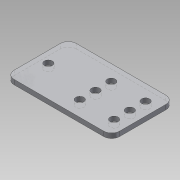
# Autodesk Inventor part: VSlot Idler Pulley Plate
Saved by Autodesk Inventor 2016 (Build 200138000, 138)
## iProperties
Created: 2013-06-20
Part Number: VSlot Idler Pulley Plate
Material: Aluminum 6061
Document SubType Name: Modeling
Designer: Jon Hollander
Density: 2.71 g/cm^3
Mass: 20.179 g
Surface Area: 59.138 cm^2
Volume: 7.44613 cm^3
Appearance: Aluminum - Flat
Author: Jon Hollander
Autodesk Inventor part; units mm, degrees
ref_plane "YZ Plane" through (0, 0, 0) normal (1, 0, 0) x (0, 1, 0)
ref_plane "XZ Plane" through (0, 0, 0) normal (0, 1, 0) x (-1, 0, 0)
ref_plane "XY Plane" through (0, 0, 0) normal (0, 0, 1) x (1, 0, 0)
sketch "Sketch2" plane through (0, 0, 0) normal (0, 0, 1) x (1, 0, 0)
  line L0 (-33.5, 19.75) -> (33.5, 19.75)
  line L1 (33.5, 19.75) -> (33.5, -19.75)
  line L2 (33.5, -19.75) -> (-33.5, -19.75)
  line L3 (-33.5, -19.75) -> (-33.5, 19.75)
  line L4 (-33.5, 19.75) -> (33.5, -19.75) construction
  line L5 (33.5, 19.75) -> (-33.5, -19.75) construction
  point P0 (0, 0)
  dimension "d0" = 67
  dimension "d1" = 39.5
  constraints: 12 end point, 2 midpoint, 2 parallel, 1 horizontal, 1 perpendicular
  measures "d0" distance of L1.end L2.end
  measures "d1" distance of L0.end L1.end
extrude "Extrusion1" add sketch "Sketch2" along normal blind 3
sketch "Sketch3" plane through (0, 0, 3) normal (0, 0, 1) x (1, 0, 0)
  line L0 (33.5, 19.75) -> (-33.5, 19.75) projected
  line L1 (-33.5, 19.75) -> (-33.5, -19.75) projected
  line L2 (-33.5, -19.75) -> (33.5, -19.75) projected
  line L3 (33.5, -19.75) -> (33.5, 19.75) projected
  line L4 (-33.5, 0) -> (33.5, 0) construction
  line L5 (3.51, 19.75) -> (3.51, -19.75) construction
  line L6 (25.29, 19.75) -> (25.29, -19.75) construction
  line L7 (-26.44, 19.75) -> (-26.44, -19.75) construction
  point P0 (0, 0)
  point P1 (-26.44, 0)
  point P2 (3.51, 0)
  point P3 (25.29, 0)
  point P4 (3.51, 10)
  point P5 (3.51, -10)
  point P6 (25.29, 10)
  point P7 (25.29, -10)
  dimension "d4" = 7.06
  dimension "d5" = 37.01
  dimension "d6" = 58.79
  dimension "d7" = 9.75
  dimension "d8" = 9.75
  dimension "d9" = 21.78
  dimension "d10" = 19.75
  constraints: 10 point on line, 8 end point, 5 midpoint, 2 horizontal alignment, 2 perpendicular, 1 vertical
  measures "d4" distance between parallel lines of L1 L7
  measures "d5" distance between parallel lines of L5 L1
  measures "d6" distance between parallel lines of L6 L1
  measures "d7" distance from line of L0 point (3.51, 10)
  measures "d8" distance from line of L2 point (3.51, -10)
  measures "d9" distance of point (25.29, 0) point (3.51, 0)
  measures "d10" distance from line of L2 point (-26.44, 0)
hole "Hole1" at (-26.44, 0, 3) at (3.51, 0, 3) at (25.29, 0, 3) at (3.51, 10, 3) at (3.51, -10, 3) at (25.29, 10, 3) at (25.29, -10, 3) direction (0, 0, -1) diameter 5.1 end through all
fillet "Fillet1" radius 5 4 edges at (33.5, 19.75, 1.5) (-33.5, 19.75, 1.5) (-33.5, -19.75, 1.5) (33.5, -19.75, 1.5)
body "Solid1"
